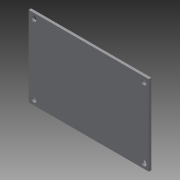
# Autodesk Inventor part: circuit
Saved by Autodesk Inventor 2013 (Build 170138000, 138)
## iProperties
Created: 2014-05-23
Part Number: circuit
Material: 一般
Document SubType Name: Modeling
Designer: andou
Density: 1 g/cm^3
Author: andou
Autodesk Inventor part; units mm, degrees
ref_plane "YZ Plane" through (0, 0, 0) normal (1, 0, 0) x (0, 1, 0)
ref_plane "XZ Plane" through (0, 0, 0) normal (0, 1, 0) x (-1, 0, 0)
ref_plane "XY Plane" through (0, 0, 0) normal (0, 0, 1) x (1, 0, 0)
sketch "スケッチ1" plane through (0, 0, 0) normal (0, 1, 0) x (-1, 0, 0)
  line L0 (-36, 24) -> (36, 24)
  line L1 (36, 24) -> (36, -24)
  line L2 (36, -24) -> (-36, -24)
  line L3 (-36, -24) -> (-36, 24)
  point P0 (0, 0)
  dimension "d0" = 72
  dimension "d2" = 48
  dimension "d3" = 24
  dimension "d4" = 36
  constraints: 8 end point, 2 parallel, 1 horizontal, 1 perpendicular
  measures "d0" distance of L0.start L0.end
  measures "d2" distance of L2.end L0.start
  measures "d3" distance from line of point (0, 0) L0
  measures "d4" distance from line of L1 point (0, 0)
extrude "押し出し1" add sketch "スケッチ1" along normal blind 1.5
sketch "スケッチ2" plane through (0, 1.5, 0) normal (0, 1, 0) x (1, 0, 0)
  line L0 (-36, -24) -> (36, -24) projected
  line L1 (36, -24) -> (36, 24) projected
  line L2 (36, 24) -> (-36, 24) projected
  line L3 (-36, 24) -> (-36, -24) projected
  circle A0 centre (-33, 21) radius 1.6
  circle A1 centre (-33, -21) radius 1.6
  circle A2 centre (33, -21) radius 1.6
  circle A3 centre (33, 21) radius 1.6
  point P0 (0, 0)
  dimension "d7" = 3.2
  dimension "d9" = 42
  dimension "d10" = 66
  dimension "d11" = 66
  dimension "d12" = 42
  dimension "d13" = 3
  dimension "d14" = 3
  dimension "d15" = 3
  dimension "d16" = 3
  constraints: 4 centre point, 3 equal radius
  measures "d7" diameter of A0
  measures "d9" distance of A1.centre A0.centre
  measures "d10" distance of A3.centre A0.centre
  measures "d11" distance of A1.centre A2.centre
  measures "d12" distance of A3.centre A2.centre
  measures "d13" distance from line of L2 A0.centre
  measures "d14" distance from line of L3 A0.centre
  measures "d15" distance from line of L2 A3.centre
  measures "d16" distance from line of L3 A1.centre
extrude "押し出し2" cut sketch "スケッチ2" against normal blind 1.5 keep common part
